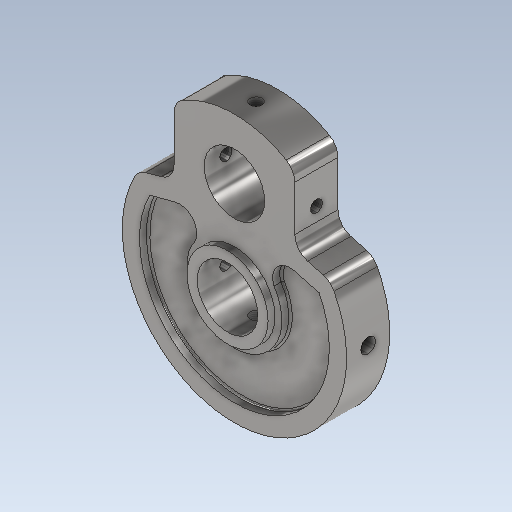
# Autodesk Inventor part: Peça15
Saved by Autodesk Inventor 2021 (Build 250183000, 183)
## iProperties
Category: 41
Created: 2021-07-18
Part Number: Peça15
Material: Liga de aço
Document SubType Name: Modeling
Designer: Giovanni
Density: 7.73 g/cm^3
Appearance: Aço - Polido
User Status: 1:2
Author: Giovanni
Keywords: 7
Autodesk Inventor part; units mm, degrees
ref_plane "XZ Plane" through (0, 0, 0) normal (0, 1, 0) x (-1, 0, 0)
ref_plane "XY Plane" through (0, 0, 0) normal (0, 0, 1) x (1, 0, 0)
sketch "Esboço1" plane through (0, 0, 0) normal (0, 0, 1) x (1, 0, 0)
  arc A0 (-55.5003, 33.8337) -> (55.5003, 33.8337) centre (0, 0) ccw
  line L0 (-35, 78.7188) -> (-35, 47)
  line L1 (-42.4118, 37.3407) -> (-55.5003, 33.8337)
  line L2 (0, 0) -> (0, 90)
  arc A1 (-42.4118, 37.3407) -> (-35, 47) centre (-45, 47) ccw
  line L3 (35, 78.7188) -> (35, 47)
  line L4 (42.4118, 37.3407) -> (55.5003, 33.8337)
  arc A2 (35, 47) -> (42.4118, 37.3407) centre (45, 47) ccw
  arc A3 (35, 78.7188) -> (-35, 78.7188) centre (0, 29.9848) ccw
  circle A4 centre (0, 0) radius 17.5
  circle A5 centre (0, 55) radius 17.5
  dimension "d1" = 65
  dimension "d3" = 35
  dimension "d4" = 105
  dimension "d5" = 10
  dimension "d6" = 47
  dimension "d7" = 10
  dimension "d8" = 35
  dimension "d9" = 105
  dimension "d10" = 60
  dimension "d11" = 90
  dimension "d12" = 35
  dimension "d13" = 55
  constraints: 10 end point, 8 point on circle, 6 centre point, 4 tangent, 3 vertical, 2 coincident, 2 horizontal alignment, 1 equal radius, 1 point on line
  measures "d1" radius of A0
  measures "d3" distance between parallel lines of L0 L2
  measures "d4" angle of L1 L0
  measures "d5" radius of A1
  measures "d6" vertical distance of point (0, 0) A1.centre
  measures "d7" radius of A2
  measures "d8" distance between parallel lines of L3 L2
  measures "d9" angle of L4 L3
  measures "d10" radius of A3
  measures "d11" distance of L2.end point (0, 0)
  measures "d12" diameter of A4
  measures "d13" distance of A5.centre point (0, 0)
extrude "Extrusão1" add sketch "Esboço1" along normal mid plane 25
sketch "Esboço5" plane through (0, 0, 12.5) normal (0, 0, 1) x (1, 0, 0)
  arc A0 (-49.1351, 24.7132) -> (49.0782, 24.826) centre (0, 0) ccw
  arc A1 (-24.8045, 11.8739) -> (22.9629, 15.1312) centre (0, 0) ccw
  arc A2 (-24.8045, 11.8739) -> (-34.4082, 28.6593) centre (-31.82, 19) ccw
  line L0 (-34.4082, 28.6593) -> (-49.1351, 24.7132)
  line L1 (-42.4118, 37.3407) -> (-55.5003, 33.8337) projected
  arc A3 (34.7724, 28.6593) -> (22.9629, 15.1312) centre (32.1842, 19) ccw
  line L2 (34.7724, 28.6593) -> (49.0782, 24.826)
  line L3 (55.5003, 33.8337) -> (42.4118, 37.3407) projected
  dimension "d21" = 55
  dimension "d22" = 27.5
  dimension "d23" = 10
  dimension "d24" = 19
  constraints: 8 point on circle, 4 centre point, 4 end point, 2 coincident, 2 parallel, 2 tangent, 1 equal radius, 1 horizontal alignment
  measures "d21" radius of A0
  measures "d22" radius of A1
  measures "d23" radius of A2
  measures "d24" vertical distance of point (0, 0) A2.centre
extrude "Extrusão2" cut sketch "Esboço5" against normal blind 5
mirror "Espelhamento1" about plane through (0, 0, 0) normal (0, 0, 1) of "Extrusão2"
sketch "Esboço6" plane through (0, 0, 12.5) normal (0, 0, 1) x (1, 0, 0)
  circle A0 centre (0, 0) radius 23.5
  circle A1 centre (0, 0) radius 17.5 projected
  dimension "d27" = 47
  constraints: 1 centre point, 1 coincident
  measures "d27" diameter of A0
extrude "Extrusão3" add sketch "Esboço6" along normal blind 4
sketch "Esboço7" plane through (0, 0, -12.5) normal (0, 0, -1) x (-1, 0, 0)
  circle A0 centre (0, 55) radius 17.5 projected
  circle A1 centre (0, 55) radius 25
  point P0 (0, 0)
  dimension "d30" = 50
  constraints: 1 centre point, 1 coincident
  measures "d30" diameter of A1
extrude "Extrusão4" add sketch "Esboço7" along normal blind 4
sketch "Esboço8" plane through (35, 47, 12.5) normal (1, 0, 0) x (0, 0, -1)
  point P0 (12.5, -47)
  point P1 (12.5, 8)
  dimension "d33" = 55
  measures "d33" distance of point (12.5, -47) point (12.5, 8)
hole "Furo1" at (35, 55, 0) direction (-1, 0, 0) diameter 6.917 depth 21.1 tip angle 118 thread size "M8x1" class "6H" standard "ANSI Metric M Profile"
pattern_circular "Padrão circular1" count 3 over 180 about axis through (0, 55, 0) along (0, 0, 1) of "Furo1"
ref_plane "Plano de trabalho1" through (65, 0, 0) normal (1, 0, 0) x (0, 1, 0)
sketch "Esboço10" plane through (65, 0, 0) normal (1, 0, 0) x (0, 1, 0)
  point P0 (0, 0)
  point P1 (0, 0)
  constraints: 1 coincident
hole "Furo2" at (65, 0, 0) direction (-1, 0, 0) diameter 8.5 depth 30
sketch "Esboço11" plane through (35, 0, 0) normal (1, 0, 0) x (0, 0, -1)
  circle A0 centre (0, 0) radius 4.25 projected
  constraints: 1 coincident
hole "Furo3" at (35, 0, 0) direction (-1, 0, 0) diameter 6.917 depth 35 thread size "M8x1" class "6H" standard "ANSI Metric M Profile"
pattern_circular "Padrão circular2" count 3 over 180 about axis through (0, 0, 0) along (0, 0, -1) of "Furo2", "Furo3"
fillet "Arredondamento1" radius 1 6 edges at (0.0632, -55, 7.5) (1.8709, -27.4363, 7.5) (41.9253, 26.7427, 7.5) (24.6509, 25.5763, 7.5) (-23.1403, 23.9661, 7.5) (-41.7717, 26.6862, 7.5)
fillet "Arredondamento2" radius 1 6 edges at (0.0632, -55, -7.5) (24.6509, 25.5763, -7.5) (41.9253, 26.7427, -7.5) (1.8709, -27.4363, -7.5) (-23.1403, 23.9661, -7.5) (-41.7717, 26.6862, -7.5)
fillet "Arredondamento3" radius 10 4 edges at (55.5003, 33.8337, 0) (35, 78.7188, 0) (-35, 78.7188, 0) (-55.5003, 33.8337, 0)
